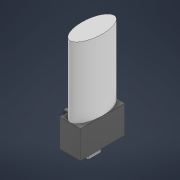
# Autodesk Inventor part: Lipo
Saved by Autodesk Inventor 2022 (Build 260153000, 153)
## iProperties
Created: 2022-03-29
Part Number: Lipo
Material: 一般
Document SubType Name: Modeling
Designer: neko2
Density: 1 g/cm^3
Appearance: 既定
Author: neko2
Autodesk Inventor part; units mm, degrees
ref_plane "YZ Plane" through (0, 0, 0) normal (1, 0, 0) x (0, 1, 0)
ref_plane "XZ Plane" through (0, 0, 0) normal (0, 1, 0) x (-1, 0, 0)
ref_plane "XY Plane" through (0, 0, 0) normal (0, 0, 1) x (1, 0, 0)
sketch "スケッチ1" plane through (0, 0, 0) normal (0, 1, 0) x (-1, 0, 0)
  line L0 (0, 0) -> (0, -12.4)
  line L1 (0, -12.4) -> (5.8, -12.4)
  line L2 (5.8, -12.4) -> (5.8, -10.2)
  line L3 (5.8, -10.2) -> (7, -10.2)
  line L4 (7, -10.2) -> (7, -9.25)
  line L5 (7, -9.25) -> (5.8, -9.25)
  line L6 (5.8, -9.25) -> (5.8, -3.15)
  line L7 (5.8, -3.15) -> (7, -3.15)
  line L8 (7, -3.15) -> (7, -2.2)
  line L9 (7, -2.2) -> (5.8, -2.2)
  line L10 (5.8, -2.2) -> (5.8, 0)
  line L11 (5.8, 0) -> (0, 0)
  dimension "d1" = 12.4
  dimension "d2" = 5.8
  dimension "d3" = 0.95
  dimension "d5" = 7
  dimension "d6" = 8
  constraints: 24 end point, 8 perpendicular, 6 point on line, 2 collinear, 1 vertical
  measures "d1" distance of L0.start L0.end
  measures "d2" distance of L0.end L1.end
  measures "d3" distance of L3.end L4.end
  measures "d5" distance between parallel lines of L0 L8
  measures "d6" distance between parallel lines of L3 L9
extrude "押し出し1" add sketch "スケッチ1" along normal blind 7.9
sketch "スケッチ2" plane through (0, 7.9, 0) normal (0, 1, 0) x (1, 0, 0)
  line L0 (-5.8, 0) -> (0, 0) projected
  line L1 (0, 12.4) -> (-5.8, 12.4) projected
  line L2 (-5.8, 12.4) -> (-5.8, 10.2) projected
  line L3 (-5.8, 10.2) -> (-7, 10.2) projected
  line L4 (-7, 10.2) -> (-7, 9.25) projected
  line L5 (-7, 9.25) -> (-5.8, 9.25) projected
  line L6 (-5.8, 9.25) -> (-5.8, 3.15) projected
  line L7 (-5.8, 3.15) -> (-7, 3.15) projected
  line L8 (-7, 3.15) -> (-7, 2.2) projected
  line L9 (-7, 2.2) -> (-5.8, 2.2) projected
  line L10 (-5.8, 2.2) -> (-5.8, 0) projected
  line L11 (-5.8, 0) -> (0, 0) projected
  line L12 (0, 0) -> (0, 12.4) projected
  ellipse E0 centre (-2.9, 6.2) end of major axis (-5.8, 6.2) minor radius 6.2
  point P0 (-2.9, 0)
  point P1 (-2.9, 12.4)
  point P2 (0, 6.2)
  point P3 (-5.8, 6.2)
  constraints: 4 midpoint, 1 vertical, 4 other
extrude "押し出し2" add sketch "スケッチ2" along normal blind 20 contours E0
sketch "スケッチ4" plane through (0, 0, 0) normal (0, -1, 0) x (1, 0, 0)
  line L0 (-2.2, -4.45) -> (-4.9, -4.45)
  line L1 (-4.9, -4.45) -> (-4.9, -7.95)
  line L2 (-4.9, -7.95) -> (-2.2, -7.95)
  line L3 (-2.2, -7.95) -> (-2.2, -4.45)
  line L4 (0, 0) -> (0, -12.4) projected
  point P0 (0, -6.2)
  point P1 (-2.2, -6.2)
  dimension "d11" = 2.7
  dimension "d12" = 3.5
  dimension "d13" = 2.2
  constraints: 8 end point, 2 midpoint, 2 parallel, 1 horizontal, 1 horizontal alignment, 1 perpendicular
  measures "d11" distance of L2.end L1.end
  measures "d12" distance of L1.end L0.end
  measures "d13" distance between parallel lines of L4 L3
extrude "押し出し3" add sketch "スケッチ4" along normal blind 3
